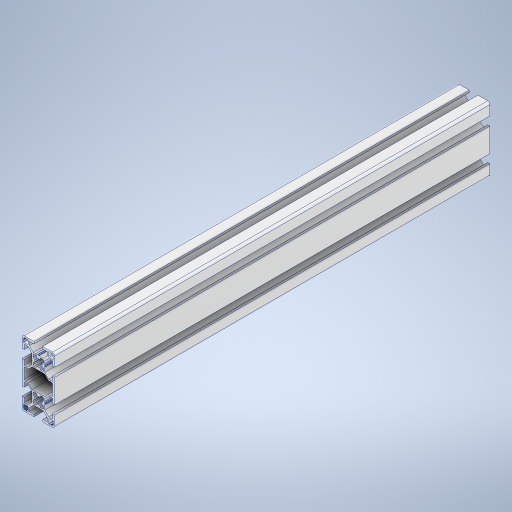
# Autodesk Inventor part: NFSL6-3060-700
Saved by Autodesk Inventor 2024 (Build 280153000, 153)
## iProperties
Category: PARTsolutions
Company: MISUMI
Created: 2024-12-13
Part Number: NFSL6-3060-700
Material: アルミニウム 6061
Catalog Web Link: www.cadenas.de
Description: NEFS6-3060, NEFSB6-3060, NEFSY6-3060, EFS6-3060, EFSB6-3060, HFS6-3060, HFSB6-3060, CAF6-3060, NFSL6-3060, HFSL6-3060, HFSLB6-3060, GFS6-3060, HFSY6-3060-Aluminum Frames -6 Series-2 Row Groove 30x60 mm Square-Specified Length
Vendor: MISUMI
Document SubType Name: Modeling
Designer: psAdmin
Manufacturer: MISUMI
Mass: 914.122 g
Surface Area: 4208.9 cm^2
Volume: 338.564 cm^3
Density: 2.7 g/cm^3
Appearance: アルミニウム - フラット
PSOL_IDENT_0: {$CADENAS_DATA/23d-libs/misumi/metric/38_al_extrusions_blackets/6/hfs6_3060.prj},757 {VTYP=3D},{NB=N
PSOL_IDENT_1: FSL6-3060-700},{LINA=NFSL6-3060-700},{NN=NEFS6-3060, NEFSB6-3060, NEFSY6-3060, EFS6-3060, EFSB6-3060
PSOL_IDENT_2: , HFS6-3060, HFSB6-3060, CAF6-3060, NFSL6-3060, HFSL6-3060, HFSLB6-3060, GFS6-3060, HFSY6-3060},{DAT
PSOL_IDENT_3: E=31.01.2024 10:05:17},{GEOMDATE=26.07.2023 02:49:00},{VERSION=},{LINEID=80},{WBVAR=L,ALT1,ALT2,ALT3
PSOL_IDENT_4: ,ALT4,ALT5,CP5,DL5,DR5,ALT6,ALT9,ALT10,ALT11,DD6SE,DD6,HP6,NHL6,DL6,NHR6,DR6,ALT7,ALT8,NH9,AH,BH,CH,
PSOL_IDENT_5: DH,EH,NH10,AV,BV,CV,DV,EV,NH11,AP,BP,CP,DP,EP,ALT12,ALT13,Z,NH12,XA,XB,XC,XD,XE,NH13,YA,YB,YC,YD,YE,
PSOL_IDENT_6: ALT14,HP14,DL14,DR14,ALT15,HP15,DL15,DR15,ALT16,HP16,DL16,DR16,ALT17,HQ17,JLP,ALT18,HQ18,KLP,ALT19,A
PSOL_IDENT_7: LT20},{WBNUMERIC=L,DD6,NH9,AH,BH,CH,DH,EH,NH10,AV,BV,CV,DV,EV,NH11,AP,BP,CP,DP,EP,NH12,XA,XB,XC,XD,X
PSOL_IDENT_8: E,NH13,YA,YB,YC,YD,YE,HQ17,JLP,HQ18,KLP}  {NB=NFSL6-3060-700},{LINA=NFSL6-3060-700},{KT=DUMMY},{PN=N
PSOL_IDENT_9: FSL6-3060-700},{TPS=NFSL6-3060},{MAT=6063-T5 Aluminum Alloy},{ST=Clear Anodize},{FRMW=30},{FRMH=60},
PSOL_IDENT_10: {FRD=6.8},{L=700.0},{MASS=1.29},{SA=476},{LX=4.87x10^4},{LY=17.87x10^4},{ALT1=},{M1=0},{IDM1=6.647},
PSOL_IDENT_11: {DALT1=4.2},{DPL1=0},{DPR1=0},{ALT1PN=},{ALT2=},{ALT2ALG= '','w/o End Tapping (Insert)','LHP','with
PSOL_IDENT_12: LHP (Tapping on the Left (Insert))','RHP','with RHP (Tapping on the Right (Insert))','HPW','with HPW
PSOL_IDENT_13: (Tapping on Both Ends (Insert))' },{M2=0},{DP2=0},{ALT2PN=},{ALT3=},{ALT3ALG= '','N/A' },{M3=0},{ID
PSOL_IDENT_14: M3=4.134},{DP3=0},{ALT3PN=},{ALT4=},{ALT4ALG= '', 'w/o SC (High Precision Cut)', 'SC', 'with SC (Hig
PSOL_IDENT_15: h Precision Cut)' },{ALT4PN=},{ALT5=},{ALT5ALG= '','w/o 45 Degree Cut','1','with 45 Degree Cut' },{C
PSOL_IDENT_16: P5=},{CP5ALG= '','N/A' },{DL5=},{DL5ALG= '','N/A' },{DR5=},{DR5ALG= '','N/A' },{FRMLALT5=0},{FRMRALT
PSOL_IDENT_17: 5=0},{ALT5PN=},{ALT6=},{ALT6ALG= '','w/o Fastening Location Wrench Access Hole Alterations','1','wit
PSOL_IDENT_18: h Fastening Location Wrench Access Hole Alterations' },{ALT9=},{ALT9ALG= '','w/o Location Specified
PSOL_IDENT_19: Wrench Access Hole Alteratons (Horizontal)','1','with Location Specified Wrench Access Hole Alterato
PSOL_IDENT_20: ns (Horizontal)' },{ALT10=},{ALT10ALG= '','w/o Location Specified Wrench Access Hole Alteratons (Ver
PSOL_IDENT_21: tical)','1','with Location Specified Wrench Access Hole Alteratons (Vertical)' },{ALT11=},{ALT11ALG=
PSOL_IDENT_22: '','w/o Location Specified Wrench Access Hole Alteratons (Crisscross)','1','with Location Specified
PSOL_IDENT_23: Wrench Access Hole Alteratons (Crisscross)' },{DD6SE=},{DD6SEALG= '','N/A' },{DD6=0},{DD6ALG=0},{HP
PSOL_IDENT_24: 6=},{HP6ALG= '','N/A' },{NHL6=},{NHL6ALG= '','N/A' },{DL6=},{DL6ALG= '','N/A' },{NHR6=},{NHR6ALG= ''
PSOL_IDENT_25: ,'N/A' },{DR6=},{DR6ALG= '','N/A' },{DD6PN=},{HL6=0},{HL6D=0},{HR6=0},{HR6D=0},{J6=0},{J6D=0},{K6=0}
PSOL_IDENT_26: ,{K6D=0},{ALT7=},{ALT7ALG= '','N/A' },{ALT8=},{ALT8ALG= '','N/A' },{ALT678PN=},{NH9=0},{NH9MAX=5},{N
PSOL_IDENT_27: H9ALG=[0]},{AH=0.0},{AHMIN=7},{AHMAX=695},{AHALG=[0]},{BH=0.0},{BHMIN=2},{BHMAX=697},{BHALG=[0]},{CH=
PSOL_IDENT_28: 0.0},{CHMIN=2},{CHMAX=699},{CHALG=[0]},{DH=0.0},{DHMIN=2},{DHMAX=701},{DHALG=[0]},{EH=0.0},{EHMIN=2}
PSOL_IDENT_29: ,{EHMAX=693},{EHALG=[0]},{NH10=0},{NH10MAX=5},{NH10ALG=[0]},{AV=0.0},{AVMIN=7},{AVMAX=695},{AVALG=[0
PSOL_IDENT_30: ]},{BV=0.0},{BVMIN=2},{BVMAX=697},{BVALG=[0]},{CV=0.0},{CVMIN=2},{CVMAX=699},{CVALG=[0]},{DV=0.0},{D
PSOL_IDENT_31: VMIN=2},{DVMAX=701},{DVALG=[0]},{EV=0.0},{EVMIN=2},{EVMAX=693},{EVALG=[0]},{NH11=0},{NH11MAX=5},{NH1
PSOL_IDENT_32: 1ALG=[0]},{AP=0.0},{APMIN=7},{APMAX=695},{APALG=[0]},{BP=0.0},{BPMIN=2},{BPMAX=697},{BPALG=[0]},{CP=
PSOL_IDENT_33: 0.0},{CPMIN=2},{CPMAX=699},{CPALG=[0]},{DP=0.0},{DPMIN=2},{DPMAX=701},{DPALG=[0]},{EP=0.0},{EPMIN=2}
PSOL_IDENT_34: ,{EPMAX=693},{EPALG=[0]},{ALT9PN=},{ALT10PN=},{ALT11PN=},{ALT91011PN=},{ALT12=},{ALT12ALG= '','w/o C
PSOL_IDENT_35: ounterbore Hole in Specified Position (Vertical)','1','with Counterbore Hole in Specified Position (
PSOL_IDENT_36: Vertical)' },{ALT13=},{ALT13ALG= '','w/o Counterbore Hole in Specified Position (Horizontal)','1','w
PSOL_IDENT_37: ith Counterbore Hole in Specified Position (Horizontal)' },{Z=},{ZALG= '','N/A' },{DD12=0.0},{DD112=
PSOL_IDENT_38: 0.0},{NH12=0},{NH12MAX=5},{NH12ALG=[0]},{XA=0.0},{XAMIN=7},{XAMAX=695},{XAALG=[0]},{XB=0.0},{XBMIN=2
PSOL_IDENT_39: },{XBMAX=697},{XBALG=[0]},{XC=0.0},{XCMIN=2},{XCMAX=699},{XCALG=[0]},{XD=0.0},{XDMIN=2},{XDMAX=701},
PSOL_IDENT_40: {XDALG=[0]},{XE=0.0},{XEMIN=2},{XEMAX=693},{XEALG=[0]},{NH13=0},{NH13MAX=5},{NH13ALG=[0]},{YA=0.0},{
PSOL_IDENT_41: YAMIN=7},{YAMAX=695},{YAALG=[0]},{YB=0.0},{YBMIN=2},{YBMAX=697},{YBALG=[0]},{YC=0.0},{YCMIN=2},{YCMA
PSOL_IDENT_42: X=699},{YCALG=[0]},{YD=0.0},{YDMIN=2},{YDMAX=701},{YDALG=[0]},{YE=0.0},{YEMIN=2},{YEMAX=693},{YEALG=
PSOL_IDENT_43: [0]},{ALT12PN=},{ALT13PN=},{ALT1213PN=},{ALT14=},{ALT14ALG= '','w/o D Type Hole Alteration','1','wit
PSOL_IDENT_44: h D Type Hole Alteration' },{HP14=},{HP14ALG= '','N/A' },{DL14=},{DL14ALG= '','N/A' },{DR14=},{DR14A
PSOL_IDENT_45: LG= '','N/A' },{H14=0},{D14=0.0},{ALT14PN=},{ALT15=},{ALT15ALG= '','w/o S Type Hole Alteration','1','
PSOL_IDENT_46: with S Type Hole Alteration' },{HP15=},{HP15ALG= '','N/A' },{DL15=},{DL15ALG= '','N/A' },{DR15=},{DR
PSOL_IDENT_47: 15ALG= '','N/A' },{H15=0},{D115=0.0},{D215=0.0},{ALT15PN=},{ALT16=},{ALT16ALG= '','w/o M Type Hole A
PSOL_IDENT_48: lteration','1','with M Type Hole Alteration' },{HP16=},{HP16ALG= '','N/A' },{DL16=},{DL16ALG= '','N/
PSOL_IDENT_49: A' },{DR16=},{DR16ALG= '','N/A' },{H116=0},{D16=0.0},{ALT16PN=},{ALT17=},{ALT17ALG= '','w/o L Type H
PSOL_IDENT_50: ole Alteration (Top)','1','with L Type Hole Alteration (Top)' },{HQ17=0},{HQ17ALG=0},{JLP=0},{JLPMIN=
PSOL_IDENT_51: 4.9},{JLPMAX=0},{JLPALG=[0]},{L17=0},{D17=0.0},{ALT18=},{ALT18ALG= '','w/o L Type Hole Alteration (B
PSOL_IDENT_52: ottom)','1','with L Type Hole Alteration (Bottom)' },{HQ18=0},{HQ18ALG=0},{KLP=0},{KLPALG=[0]},{KLPM
PSOL_IDENT_53: IN=4.9},{KLPMAX=0},{L18=0},{D18=0.0},{ALT19=},{ALT19ALG= '','N/A' },{M19=0},{DP19=0},{ALT1718PN=},{A
PSOL_IDENT_54: LT19PN=},{ALT20=},{ALT20PN=},{ERRORALT01=OK},{ERRORALT02=OK},{ERRORALT03=OK},{ERRORALT05=OK},{ERRORA
PSOL_IDENT_55: LT06091=OK},{ERRORALT06092=OK},{ERRORALT06093=OK},{ERRORALT06094=OK},{ERRORALT06101=OK},{ERRORALT061
PSOL_IDENT_56: 02=OK},{ERRORALT06103=OK},{ERRORALT06104=OK},{ERRORALT06111=OK},{ERRORALT06112=OK},{ERRORALT06113=OK
PSOL_IDENT_57: },{ERRORALT06114=OK},{ERRORALT06121=OK},{ERRORALT06122=OK},{ERRORALT06123=OK},{ERRORALT06124=OK},{ER
PSOL_IDENT_58: RORALT06131=OK},{ERRORALT06132=OK},{ERRORALT06133=OK},{ERRORALT06134=OK},{ERRORALT0614=OK},{ERRORALT
PSOL_IDENT_59: 0615=OK},{ERRORALT0616=OK},{ERRORALT06171=OK},{ERRORALT06172=OK},{ERRORALT06173=OK},{ERRORALT06181=O
PSOL_IDENT_60: K},{ERRORALT06182=OK},{ERRORALT06183=OK},{ERRORALT0619=OK},{ERRORALT0911=OK},{ERRORALT0913=OK},{ERRO
PSOL_IDENT_61: RALT0914=OK},{ERRORALT0915=OK},{ERRORALT0916=OK},{ERRORALT0917=OK},{ERRORALT0918=OK},{ERRORALT0919=O
PSOL_IDENT_62: K},{ERRORALT1011=OK},{ERRORALT1012=OK},{ERRORALT1014=OK},{ERRORALT1015=OK},{ERRORALT1016=OK},{ERRORA
PSOL_IDENT_63: LT1017=OK},{ERRORALT1018=OK},{ERRORALT1019=OK},{ERRORALT1112=OK},{ERRORALT1113=OK},{ERRORALT1114=OK}
PSOL_IDENT_64: ,{ERRORALT1115=OK},{ERRORALT1116=OK},{ERRORALT1117=OK},{ERRORALT1118=OK},{ERRORALT1119=OK},{ERRORALT
PSOL_IDENT_65: 1214=OK},{ERRORALT1215=OK},{ERRORALT1216=OK},{ERRORALT1217=OK},{ERRORALT1218=OK},{ERRORALT1219=OK},{
PSOL_IDENT_66: ERRORALT1314=OK},{ERRORALT1315=OK},{ERRORALT1316=OK},{ERRORALT1317=OK},{ERRORALT1318=OK},{ERRORALT13
PSOL_IDENT_67: 19=OK},{ERRORALT1415=OK},{ERRORALT1416=OK},{ERRORALT1417=OK},{ERRORALT1418=OK},{ERRORALT1419=OK},{ER
PSOL_IDENT_68: RORALT1516=OK},{ERRORALT1517=OK},{ERRORALT1518=OK},{ERRORALT1519=OK},{ERRORALT1617=OK},{ERRORALT1618=
PSOL_IDENT_69: OK},{ERRORALT1619=OK},{ERRORALT1719=OK},{ERRORALT1819=OK},{ERRORPN=},{COLOR=}
NB: NFSL6-3060-700
NN: NEFS6-3060, NEFSB6-3060, NEFSY6-3060, EFS6-3060, EFSB6-3060, HFS6-3060, HFSB6-3060, CAF6-3060, NFSL6-3060, HFSL6-3060, HFSLB6-3060, GFS6-3060, HFSY6-3060
NT: Aluminum Frames -6 Series-2 Row Groove 30x60 mm Square-Specified Length
NBSYN: $PN.
LINA: NFSL6-3060-700
CATALOG: Misumi
PN: NFSL6-3060-700
TPS: NFSL6-3060
MAT: 6063-T5 Aluminum Alloy
ST: Clear Anodize
L: 700
MASS: 1.29
SA: 476
LX: 4.87x10^4
LY: 17.87x10^4
ALT1: w/o End Tapping
DPL1: 0
DPR1: 0
ALT2: w/o End Tapping (Insert)
M2: 0
DP2: 0
ALT3: N/A
M3: 0
DP3: 0
ALT4: w/o SC (High Precision Cut)
ALT5: w/o 45 Degree Cut
CP5: N/A
DL5: N/A
DR5: N/A
ALT6: w/o Fastening Location Wrench Access Hole Alterations
ALT9: w/o Location Specified Wrench Access Hole Alteratons (Horizontal)
ALT10: w/o Location Specified Wrench Access Hole Alteratons (Vertical)
ALT11: w/o Location Specified Wrench Access Hole Alteratons (Crisscross)
DD6SE: N/A
DD6: 0
HP6: N/A
NHL6: N/A
DL6: N/A
NHR6: N/A
DR6: N/A
HL6D: 0
HR6D: 0
J6D: 0
K6D: 0
ALT7: N/A
ALT8: N/A
NH9: 0
AH: 0
BH: 0
CH: 0
DH: 0
EH: 0
NH10: 0
AV: 0
BV: 0
CV: 0
DV: 0
EV: 0
NH11: 0
AP: 0
BP: 0
CP: 0
DP: 0
EP: 0
ALT12: w/o Counterbore Hole in Specified Position (Vertical)
ALT13: w/o Counterbore Hole in Specified Position (Horizontal)
Z: N/A
DD12: 0
DD112: 0
NH12: 0
XA: 0
XB: 0
XC: 0
XD: 0
XE: 0
NH13: 0
YA: 0
YB: 0
YC: 0
YD: 0
YE: 0
ALT14: w/o D Type Hole Alteration
HP14: N/A
DL14: N/A
DR14: N/A
H14: 0
D14: 0
ALT15: w/o S Type Hole Alteration
HP15: N/A
DL15: N/A
DR15: N/A
H15: 0
D115: 0
D215: 0
ALT16: w/o M Type Hole Alteration
HP16: N/A
DL16: N/A
DR16: N/A
H116: 0
D16: 0
ALT17: w/o L Type Hole Alteration (Top)
HQ17: 0
JLP: 0
D17: 0
ALT18: w/o L Type Hole Alteration (Bottom)
HQ18: 0
KLP: 0
D18: 0
ALT19: N/A
M19: 0
DP19: 0
ALT20: w/o CW (End Face C Chamfering)
SUPPLIER: MISUMI
ARTICLENO: NFSL6-3060-700
BOMINFO: NFSL6-3060-700
CREATOR: CADENAS GmbH
Title: NFSL6-3060-700
Author: Cadenas PARTsolutions
Comments: Aluminum Frames -6 Series-2 Row Groove 30x60 mm Square-Specified Length
Autodesk Inventor part; units mm, degrees
sketch "Sketch_118" plane through (0, 0, 0) normal (0, 0, 1) x (1, 0, 0)
  line L0 (-15, 11) -> (-15, -11)
  line L1 (-15, -11) -> (-13, -11)
  line L2 (-13, -11) -> (-13, -6.75)
  line L3 (-13, -6.75) -> (-9.6642, -6.75)
  line L4 (-9.6642, -6.75) -> (-6, -10.4142)
  line L5 (-6, -10.4142) -> (-6, -14.3464)
  arc A0 (-6, -14.3464) -> (-5.933, -14.5964) centre (-5.5, -14.3464) ccw
  line L6 (-5.933, -14.5964) -> (-5.7, -15)
  line L7 (-5.7, -15) -> (-5.933, -15.4036)
  arc A1 (-5.933, -15.4036) -> (-5.933, -15.9036) centre (-5.5, -15.6536) ccw
  line L8 (-5.933, -15.9036) -> (-5.751, -16.2189)
  line L9 (-5.751, -16.2189) -> (-6, -17.5)
  line L10 (-6, -17.5) -> (-6, -19.5858)
  line L11 (-6, -19.5858) -> (-9.6642, -23.25)
  line L12 (-9.6642, -23.25) -> (-13, -23.25)
  line L13 (-13, -23.25) -> (-13, -19)
  line L14 (-13, -19) -> (-15, -19)
  line L15 (-15, -19) -> (-15, -28)
  arc A2 (-15, -28) -> (-13, -30) centre (-13, -28) ccw
  line L16 (-13, -30) -> (-4, -30)
  line L17 (-4, -30) -> (-4, -28)
  line L18 (-4, -28) -> (-8.25, -28)
  line L19 (-8.25, -28) -> (-8.25, -24.6642)
  line L20 (-8.25, -24.6642) -> (-4.5858, -21)
  line L21 (-4.5858, -21) -> (-0.6536, -21)
  arc A3 (-0.6536, -21) -> (-0.4036, -20.933) centre (-0.6536, -20.5) ccw
  line L22 (-0.4036, -20.933) -> (0, -20.7)
  line L23 (0, -20.7) -> (0.4036, -20.933)
  arc A4 (0.4036, -20.933) -> (0.9036, -20.933) centre (0.6536, -20.5) ccw
  line L24 (0.9036, -20.933) -> (1.2189, -20.751)
  line L25 (1.2189, -20.751) -> (2.5, -21)
  line L26 (2.5, -21) -> (4.5858, -21)
  line L27 (4.5858, -21) -> (8.25, -24.6642)
  line L28 (8.25, -24.6642) -> (8.25, -28)
  line L29 (8.25, -28) -> (4, -28)
  line L30 (4, -28) -> (4, -30)
  line L31 (4, -30) -> (13, -30)
  arc A5 (13, -30) -> (15, -28) centre (13, -28) ccw
  line L32 (15, -28) -> (15, -19)
  line L33 (15, -19) -> (13, -19)
  line L34 (13, -19) -> (13, -23.25)
  line L35 (13, -23.25) -> (9.6642, -23.25)
  line L36 (9.6642, -23.25) -> (6, -19.5858)
  line L37 (6, -19.5858) -> (6, -15.6536)
  arc A6 (6, -15.6536) -> (5.933, -15.4036) centre (5.5, -15.6536) ccw
  line L38 (5.933, -15.4036) -> (5.7, -15)
  line L39 (5.7, -15) -> (5.933, -14.5964)
  arc A7 (5.933, -14.5964) -> (5.933, -14.0964) centre (5.5, -14.3464) ccw
  line L40 (5.933, -14.0964) -> (5.751, -13.7811)
  line L41 (5.751, -13.7811) -> (6, -12.5)
  line L42 (6, -12.5) -> (6, -10.4142)
  line L43 (6, -10.4142) -> (9.6642, -6.75)
  line L44 (9.6642, -6.75) -> (13, -6.75)
  line L45 (13, -6.75) -> (13, -11)
  line L46 (13, -11) -> (15, -11)
  line L47 (15, -11) -> (15, 11)
  line L48 (15, 11) -> (13, 11)
  line L49 (13, 11) -> (13, 6.75)
  line L50 (13, 6.75) -> (9.6642, 6.75)
  line L51 (9.6642, 6.75) -> (6, 10.4142)
  line L52 (6, 10.4142) -> (6, 14.3464)
  arc A8 (6, 14.3464) -> (5.933, 14.5964) centre (5.5, 14.3464) ccw
  line L53 (5.933, 14.5964) -> (5.7, 15)
  line L54 (5.7, 15) -> (5.933, 15.4036)
  arc A9 (5.933, 15.4036) -> (5.933, 15.9036) centre (5.5, 15.6536) ccw
  line L55 (5.933, 15.9036) -> (5.751, 16.2189)
  line L56 (5.751, 16.2189) -> (6, 17.5)
  line L57 (6, 17.5) -> (6, 19.5858)
  line L58 (6, 19.5858) -> (9.6642, 23.25)
  line L59 (9.6642, 23.25) -> (13, 23.25)
  line L60 (13, 23.25) -> (13, 19)
  line L61 (13, 19) -> (15, 19)
  line L62 (15, 19) -> (15, 28)
  arc A10 (15, 28) -> (13, 30) centre (13, 28) ccw
  line L63 (13, 30) -> (4, 30)
  line L64 (4, 30) -> (4, 28)
  line L65 (4, 28) -> (8.25, 28)
  line L66 (8.25, 28) -> (8.25, 24.6642)
  line L67 (8.25, 24.6642) -> (4.5858, 21)
  line L68 (4.5858, 21) -> (0.6536, 21)
  arc A11 (0.6536, 21) -> (0.4036, 20.933) centre (0.6536, 20.5) ccw
  line L69 (0.4036, 20.933) -> (0, 20.7)
  line L70 (0, 20.7) -> (-0.4036, 20.933)
  arc A12 (-0.4036, 20.933) -> (-0.9036, 20.933) centre (-0.6536, 20.5) ccw
  line L71 (-0.9036, 20.933) -> (-1.2189, 20.751)
  line L72 (-1.2189, 20.751) -> (-2.5, 21)
  line L73 (-2.5, 21) -> (-4.5858, 21)
  line L74 (-4.5858, 21) -> (-8.25, 24.6642)
  line L75 (-8.25, 24.6642) -> (-8.25, 28)
  line L76 (-8.25, 28) -> (-4, 28)
  line L77 (-4, 28) -> (-4, 30)
  line L78 (-4, 30) -> (-13, 30)
  arc A13 (-13, 30) -> (-15, 28) centre (-13, 28) ccw
  line L79 (-15, 28) -> (-15, 19)
  line L80 (-15, 19) -> (-13, 19)
  line L81 (-13, 19) -> (-13, 23.25)
  line L82 (-13, 23.25) -> (-9.6642, 23.25)
  line L83 (-9.6642, 23.25) -> (-6, 19.5858)
  line L84 (-6, 19.5858) -> (-6, 15.6536)
  arc A14 (-6, 15.6536) -> (-5.933, 15.4036) centre (-5.5, 15.6536) ccw
  line L85 (-5.933, 15.4036) -> (-5.7, 15)
  line L86 (-5.7, 15) -> (-5.933, 14.5964)
  arc A15 (-5.933, 14.5964) -> (-5.933, 14.0964) centre (-5.5, 14.3464) ccw
  line L87 (-5.933, 14.0964) -> (-5.751, 13.7811)
  line L88 (-5.751, 13.7811) -> (-6, 12.5)
  line L89 (-6, 12.5) -> (-6, 10.4142)
  line L90 (-6, 10.4142) -> (-9.6642, 6.75)
  line L91 (-9.6642, 6.75) -> (-13, 6.75)
  line L92 (-13, 6.75) -> (-13, 11)
  line L93 (-13, 11) -> (-15, 11)
  line L94 (9.5, 28.6) -> (9.5, 25)
  arc A16 (9.5, 25) -> (10, 24.5) centre (10, 25) ccw
  line L95 (10, 24.5) -> (13.6, 24.5)
  arc A17 (13.6, 24.5) -> (13.8, 24.7) centre (13.6, 24.7) ccw
  line L96 (13.8, 24.7) -> (13.8, 26.2)
  arc A18 (13.8, 26.2) -> (13.6, 26.4) centre (13.6, 26.2) ccw
  line L97 (13.6, 26.4) -> (13.43, 26.4)
  arc A19 (13.23, 26.6) -> (13.43, 26.4) centre (13.43, 26.6) ccw
  line L98 (13.23, 26.6) -> (13.23, 27)
  arc A20 (13.43, 27.2) -> (13.23, 27) centre (13.43, 27) ccw
  line L99 (13.43, 27.2) -> (13.6, 27.2)
  arc A21 (13.6, 27.2) -> (13.8, 27.4) centre (13.6, 27.4) ccw
  line L100 (13.8, 27.4) -> (13.8, 27.6)
  arc A22 (13.8, 27.6) -> (13.5, 27.9) centre (13.5, 27.6) ccw
  line L101 (13.5, 27.9) -> (13.2, 27.9)
  arc A23 (12.9, 28.2) -> (13.2, 27.9) centre (13.2, 28.2) ccw
  line L102 (12.9, 28.2) -> (12.9, 28.5)
  arc A24 (12.9, 28.5) -> (12.6, 28.8) centre (12.6, 28.5) ccw
  line L103 (12.6, 28.8) -> (12.4, 28.8)
  arc A25 (12.4, 28.8) -> (12.2, 28.6) centre (12.4, 28.6) ccw
  line L104 (12.2, 28.6) -> (12.2, 28.43)
  arc A26 (12, 28.23) -> (12.2, 28.43) centre (12, 28.43) ccw
  line L105 (12, 28.23) -> (11.6, 28.23)
  arc A27 (11.4, 28.43) -> (11.6, 28.23) centre (11.6, 28.43) ccw
  line L106 (11.4, 28.43) -> (11.4, 28.6)
  arc A28 (11.4, 28.6) -> (11.2, 28.8) centre (11.2, 28.6) ccw
  line L107 (11.2, 28.8) -> (9.7, 28.8)
  arc A29 (9.7, 28.8) -> (9.5, 28.6) centre (9.7, 28.6) ccw
  arc A30 (9.5, -28.6) -> (9.7, -28.8) centre (9.7, -28.6) ccw
  line L108 (9.7, -28.8) -> (11.2, -28.8)
  arc A31 (11.2, -28.8) -> (11.4, -28.6) centre (11.2, -28.6) ccw
  line L109 (11.4, -28.6) -> (11.4, -28.43)
  arc A32 (11.6, -28.23) -> (11.4, -28.43) centre (11.6, -28.43) ccw
  line L110 (11.6, -28.23) -> (12, -28.23)
  arc A33 (12.2, -28.43) -> (12, -28.23) centre (12, -28.43) ccw
  line L111 (12.2, -28.43) -> (12.2, -28.6)
  arc A34 (12.2, -28.6) -> (12.4, -28.8) centre (12.4, -28.6) ccw
  line L112 (12.4, -28.8) -> (12.6, -28.8)
  arc A35 (12.6, -28.8) -> (12.9, -28.5) centre (12.6, -28.5) ccw
  line L113 (12.9, -28.5) -> (12.9, -28.2)
  arc A36 (13.2, -27.9) -> (12.9, -28.2) centre (13.2, -28.2) ccw
  line L114 (13.2, -27.9) -> (13.5, -27.9)
  arc A37 (13.5, -27.9) -> (13.8, -27.6) centre (13.5, -27.6) ccw
  line L115 (13.8, -27.6) -> (13.8, -27.4)
  arc A38 (13.8, -27.4) -> (13.6, -27.2) centre (13.6, -27.4) ccw
  line L116 (13.6, -27.2) -> (13.43, -27.2)
  arc A39 (13.23, -27) -> (13.43, -27.2) centre (13.43, -27) ccw
  line L117 (13.23, -27) -> (13.23, -26.6)
  arc A40 (13.43, -26.4) -> (13.23, -26.6) centre (13.43, -26.6) ccw
  line L118 (13.43, -26.4) -> (13.6, -26.4)
  arc A41 (13.6, -26.4) -> (13.8, -26.2) centre (13.6, -26.2) ccw
  line L119 (13.8, -26.2) -> (13.8, -24.7)
  arc A42 (13.8, -24.7) -> (13.6, -24.5) centre (13.6, -24.7) ccw
  line L120 (13.6, -24.5) -> (10, -24.5)
  arc A43 (10, -24.5) -> (9.5, -25) centre (10, -25) ccw
  line L121 (9.5, -25) -> (9.5, -28.6)
  arc A44 (-13, -4.55) -> (-12, -5.55) centre (-12, -4.55) ccw
  line L122 (-12, -5.55) -> (-9.1672, -5.55)
  line L123 (-9.1672, -5.55) -> (-5.7172, -9)
  line L124 (-5.7172, -9) -> (5.7172, -9)
  line L125 (5.7172, -9) -> (9.1672, -5.55)
  line L126 (9.1672, -5.55) -> (12, -5.55)
  arc A45 (12, -5.55) -> (13, -4.55) centre (12, -4.55) ccw
  line L127 (13, -4.55) -> (13, 4.55)
  arc A46 (13, 4.55) -> (12, 5.55) centre (12, 4.55) ccw
  line L128 (12, 5.55) -> (9.1672, 5.55)
  line L129 (9.1672, 5.55) -> (5.7172, 9)
  line L130 (5.7172, 9) -> (-5.7172, 9)
  line L131 (-5.7172, 9) -> (-9.1672, 5.55)
  line L132 (-9.1672, 5.55) -> (-12, 5.55)
  arc A47 (-12, 5.55) -> (-13, 4.55) centre (-12, 4.55) ccw
  line L133 (-13, 4.55) -> (-13, -4.55)
  line L134 (-13.8, 26.2) -> (-13.8, 24.7)
  arc A48 (-13.8, 24.7) -> (-13.6, 24.5) centre (-13.6, 24.7) ccw
  line L135 (-13.6, 24.5) -> (-10, 24.5)
  arc A49 (-10, 24.5) -> (-9.5, 25) centre (-10, 25) ccw
  line L136 (-9.5, 25) -> (-9.5, 28.6)
  arc A50 (-9.5, 28.6) -> (-9.7, 28.8) centre (-9.7, 28.6) ccw
  line L137 (-9.7, 28.8) -> (-11.2, 28.8)
  arc A51 (-11.2, 28.8) -> (-11.4, 28.6) centre (-11.2, 28.6) ccw
  line L138 (-11.4, 28.6) -> (-11.4, 28.43)
  arc A52 (-11.6, 28.23) -> (-11.4, 28.43) centre (-11.6, 28.43) ccw
  line L139 (-11.6, 28.23) -> (-12, 28.23)
  arc A53 (-12.2, 28.43) -> (-12, 28.23) centre (-12, 28.43) ccw
  line L140 (-12.2, 28.43) -> (-12.2, 28.6)
  arc A54 (-12.2, 28.6) -> (-12.4, 28.8) centre (-12.4, 28.6) ccw
  line L141 (-12.4, 28.8) -> (-12.6, 28.8)
  arc A55 (-12.6, 28.8) -> (-12.9, 28.5) centre (-12.6, 28.5) ccw
  line L142 (-12.9, 28.5) -> (-12.9, 28.2)
  arc A56 (-13.2, 27.9) -> (-12.9, 28.2) centre (-13.2, 28.2) ccw
  line L143 (-13.2, 27.9) -> (-13.5, 27.9)
  arc A57 (-13.5, 27.9) -> (-13.8, 27.6) centre (-13.5, 27.6) ccw
  line L144 (-13.8, 27.6) -> (-13.8, 27.4)
  arc A58 (-13.8, 27.4) -> (-13.6, 27.2) centre (-13.6, 27.4) ccw
  line L145 (-13.6, 27.2) -> (-13.43, 27.2)
  arc A59 (-13.23, 27) -> (-13.43, 27.2) centre (-13.43, 27) ccw
  line L146 (-13.23, 27) -> (-13.23, 26.6)
  arc A60 (-13.43, 26.4) -> (-13.23, 26.6) centre (-13.43, 26.6) ccw
  line L147 (-13.43, 26.4) -> (-13.6, 26.4)
  arc A61 (-13.6, 26.4) -> (-13.8, 26.2) centre (-13.6, 26.2) ccw
  arc A62 (-13.8, -26.2) -> (-13.6, -26.4) centre (-13.6, -26.2) ccw
  line L148 (-13.6, -26.4) -> (-13.43, -26.4)
  arc A63 (-13.23, -26.6) -> (-13.43, -26.4) centre (-13.43, -26.6) ccw
  line L149 (-13.23, -26.6) -> (-13.23, -27)
  arc A64 (-13.43, -27.2) -> (-13.23, -27) centre (-13.43, -27) ccw
  line L150 (-13.43, -27.2) -> (-13.6, -27.2)
  arc A65 (-13.6, -27.2) -> (-13.8, -27.4) centre (-13.6, -27.4) ccw
  line L151 (-13.8, -27.4) -> (-13.8, -27.6)
  arc A66 (-13.8, -27.6) -> (-13.5, -27.9) centre (-13.5, -27.6) ccw
  line L152 (-13.5, -27.9) -> (-13.2, -27.9)
  arc A67 (-12.9, -28.2) -> (-13.2, -27.9) centre (-13.2, -28.2) ccw
  line L153 (-12.9, -28.2) -> (-12.9, -28.5)
  arc A68 (-12.9, -28.5) -> (-12.6, -28.8) centre (-12.6, -28.5) ccw
  line L154 (-12.6, -28.8) -> (-12.4, -28.8)
  arc A69 (-12.4, -28.8) -> (-12.2, -28.6) centre (-12.4, -28.6) ccw
  line L155 (-12.2, -28.6) -> (-12.2, -28.43)
  arc A70 (-12, -28.23) -> (-12.2, -28.43) centre (-12, -28.43) ccw
  line L156 (-12, -28.23) -> (-11.6, -28.23)
  arc A71 (-11.4, -28.43) -> (-11.6, -28.23) centre (-11.6, -28.43) ccw
  line L157 (-11.4, -28.43) -> (-11.4, -28.6)
  arc A72 (-11.4, -28.6) -> (-11.2, -28.8) centre (-11.2, -28.6) ccw
  line L158 (-11.2, -28.8) -> (-9.7, -28.8)
  arc A73 (-9.7, -28.8) -> (-9.5, -28.6) centre (-9.7, -28.6) ccw
  line L159 (-9.5, -28.6) -> (-9.5, -25)
  arc A74 (-9.5, -25) -> (-10, -24.5) centre (-10, -25) ccw
  line L160 (-10, -24.5) -> (-13.6, -24.5)
  arc A75 (-13.6, -24.5) -> (-13.8, -24.7) centre (-13.6, -24.7) ccw
  line L161 (-13.8, -24.7) -> (-13.8, -26.2)
  constraints: 324 end point, 152 point on circle, 76 centre point
extrude "Extrusion1" add sketch "Sketch_118" against normal blind 400
sketch "Sketch_94" plane through (0, 0, 0) normal (0, 0, 1) x (1, 0, 0)
  line L0 (-4.8, 18.8) -> (-4.8, 17.2312)
  arc A0 (-4.8, 17.2312) -> (-4.4833, 16.766) centre (-4.3, 17.2312) ccw
  line L1 (-4.4833, 16.766) -> (-3.5987, 16.4176)
  arc A1 (-3.2971, 15.8303) -> (-3.5987, 16.4176) centre (-3.7819, 15.9524) ccw
  arc A2 (-3.2971, 15.8303) -> (-3.4, 15) centre (0, 15) ccw
  arc A3 (-3.4, 15) -> (-3.2971, 14.1697) centre (0, 15) ccw
  arc A4 (-3.5987, 13.5824) -> (-3.2971, 14.1697) centre (-3.7819, 14.0476) ccw
  line L2 (-3.5987, 13.5824) -> (-4.4833, 13.234)
  arc A5 (-4.4833, 13.234) -> (-4.8, 12.7688) centre (-4.3, 12.7688) ccw
  line L3 (-4.8, 12.7688) -> (-4.8, 11.2)
  arc A6 (-4.8, 11.2) -> (-3.8, 10.2) centre (-3.8, 11.2) ccw
  line L4 (-3.8, 10.2) -> (-2.2312, 10.2)
  arc A7 (-2.2312, 10.2) -> (-1.766, 10.5167) centre (-2.2312, 10.7) ccw
  line L5 (-1.766, 10.5167) -> (-1.4176, 11.4013)
  arc A8 (-0.8303, 11.7029) -> (-1.4176, 11.4013) centre (-0.9524, 11.2181) ccw
  arc A9 (-0.8303, 11.7029) -> (0, 11.6) centre (0, 15) ccw
  arc A10 (0, 11.6) -> (0.8303, 11.7029) centre (0, 15) ccw
  arc A11 (1.4176, 11.4013) -> (0.8303, 11.7029) centre (0.9524, 11.2181) ccw
  line L6 (1.4176, 11.4013) -> (1.766, 10.5167)
  arc A12 (1.766, 10.5167) -> (2.2312, 10.2) centre (2.2312, 10.7) ccw
  line L7 (2.2312, 10.2) -> (3.8, 10.2)
  arc A13 (3.8, 10.2) -> (4.8, 11.2) centre (3.8, 11.2) ccw
  line L8 (4.8, 11.2) -> (4.8, 12.7688)
  arc A14 (4.8, 12.7688) -> (4.4833, 13.234) centre (4.3, 12.7688) ccw
  line L9 (4.4833, 13.234) -> (3.5987, 13.5824)
  arc A15 (3.2971, 14.1697) -> (3.5987, 13.5824) centre (3.7819, 14.0476) ccw
  arc A16 (3.2971, 14.1697) -> (3.4, 15) centre (0, 15) ccw
  arc A17 (3.4, 15) -> (3.2971, 15.8303) centre (0, 15) ccw
  arc A18 (3.5987, 16.4176) -> (3.2971, 15.8303) centre (3.7819, 15.9524) ccw
  line L10 (3.5987, 16.4176) -> (4.4833, 16.766)
  arc A19 (4.4833, 16.766) -> (4.8, 17.2312) centre (4.3, 17.2312) ccw
  line L11 (4.8, 17.2312) -> (4.8, 18.8)
  arc A20 (4.8, 18.8) -> (3.8, 19.8) centre (3.8, 18.8) ccw
  line L12 (3.8, 19.8) -> (2.2312, 19.8)
  arc A21 (2.2312, 19.8) -> (1.766, 19.4833) centre (2.2312, 19.3) ccw
  line L13 (1.766, 19.4833) -> (1.4176, 18.5987)
  arc A22 (0.8303, 18.2971) -> (1.4176, 18.5987) centre (0.9524, 18.7819) ccw
  arc A23 (0.8303, 18.2971) -> (0, 18.4) centre (0, 15) ccw
  arc A24 (0, 18.4) -> (-0.8303, 18.2971) centre (0, 15) ccw
  arc A25 (-1.4176, 18.5987) -> (-0.8303, 18.2971) centre (-0.9524, 18.7819) ccw
  line L14 (-1.4176, 18.5987) -> (-1.766, 19.4833)
  arc A26 (-1.766, 19.4833) -> (-2.2312, 19.8) centre (-2.2312, 19.3) ccw
  line L15 (-2.2312, 19.8) -> (-3.8, 19.8)
  arc A27 (-3.8, 19.8) -> (-4.8, 18.8) centre (-3.8, 18.8) ccw
  constraints: 56 point on circle, 32 end point, 28 centre point
extrude "Extrusion2" cut sketch "Sketch_94" against normal blind 700
sketch "Sketch_113" plane through (0, 0, 0) normal (0, 0, 1) x (1, 0, 0)
  arc A0 (-4.8, -18.8) -> (-3.8, -19.8) centre (-3.8, -18.8) ccw
  line L0 (-3.8, -19.8) -> (-2.2312, -19.8)
  arc A1 (-2.2312, -19.8) -> (-1.766, -19.4833) centre (-2.2312, -19.3) ccw
  line L1 (-1.766, -19.4833) -> (-1.4176, -18.5987)
  arc A2 (-0.8303, -18.2971) -> (-1.4176, -18.5987) centre (-0.9524, -18.7819) ccw
  arc A3 (-0.8303, -18.2971) -> (0, -18.4) centre (0, -15) ccw
  arc A4 (0, -18.4) -> (0.8303, -18.2971) centre (0, -15) ccw
  arc A5 (1.4176, -18.5987) -> (0.8303, -18.2971) centre (0.9524, -18.7819) ccw
  line L2 (1.4176, -18.5987) -> (1.766, -19.4833)
  arc A6 (1.766, -19.4833) -> (2.2312, -19.8) centre (2.2312, -19.3) ccw
  line L3 (2.2312, -19.8) -> (3.8, -19.8)
  arc A7 (3.8, -19.8) -> (4.8, -18.8) centre (3.8, -18.8) ccw
  line L4 (4.8, -18.8) -> (4.8, -17.2312)
  arc A8 (4.8, -17.2312) -> (4.4833, -16.766) centre (4.3, -17.2312) ccw
  line L5 (4.4833, -16.766) -> (3.5987, -16.4176)
  arc A9 (3.2971, -15.8303) -> (3.5987, -16.4176) centre (3.7819, -15.9524) ccw
  arc A10 (3.2971, -15.8303) -> (3.4, -15) centre (0, -15) ccw
  arc A11 (3.4, -15) -> (3.2971, -14.1697) centre (0, -15) ccw
  arc A12 (3.5987, -13.5824) -> (3.2971, -14.1697) centre (3.7819, -14.0476) ccw
  line L6 (3.5987, -13.5824) -> (4.4833, -13.234)
  arc A13 (4.4833, -13.234) -> (4.8, -12.7688) centre (4.3, -12.7688) ccw
  line L7 (4.8, -12.7688) -> (4.8, -11.2)
  arc A14 (4.8, -11.2) -> (3.8, -10.2) centre (3.8, -11.2) ccw
  line L8 (3.8, -10.2) -> (2.2312, -10.2)
  arc A15 (2.2312, -10.2) -> (1.766, -10.5167) centre (2.2312, -10.7) ccw
  line L9 (1.766, -10.5167) -> (1.4176, -11.4013)
  arc A16 (0.8303, -11.7029) -> (1.4176, -11.4013) centre (0.9524, -11.2181) ccw
  arc A17 (0.8303, -11.7029) -> (0, -11.6) centre (0, -15) ccw
  arc A18 (0, -11.6) -> (-0.8303, -11.7029) centre (0, -15) ccw
  arc A19 (-1.4176, -11.4013) -> (-0.8303, -11.7029) centre (-0.9524, -11.2181) ccw
  line L10 (-1.4176, -11.4013) -> (-1.766, -10.5167)
  arc A20 (-1.766, -10.5167) -> (-2.2312, -10.2) centre (-2.2312, -10.7) ccw
  line L11 (-2.2312, -10.2) -> (-3.8, -10.2)
  arc A21 (-3.8, -10.2) -> (-4.8, -11.2) centre (-3.8, -11.2) ccw
  line L12 (-4.8, -11.2) -> (-4.8, -12.7688)
  arc A22 (-4.8, -12.7688) -> (-4.4833, -13.234) centre (-4.3, -12.7688) ccw
  line L13 (-4.4833, -13.234) -> (-3.5987, -13.5824)
  arc A23 (-3.2971, -14.1697) -> (-3.5987, -13.5824) centre (-3.7819, -14.0476) ccw
  arc A24 (-3.2971, -14.1697) -> (-3.4, -15) centre (0, -15) ccw
  arc A25 (-3.4, -15) -> (-3.2971, -15.8303) centre (0, -15) ccw
  arc A26 (-3.5987, -16.4176) -> (-3.2971, -15.8303) centre (-3.7819, -15.9524) ccw
  line L14 (-3.5987, -16.4176) -> (-4.4833, -16.766)
  arc A27 (-4.4833, -16.766) -> (-4.8, -17.2312) centre (-4.3, -17.2312) ccw
  line L15 (-4.8, -17.2312) -> (-4.8, -18.8)
  constraints: 56 point on circle, 32 end point, 28 centre point
extrude "Extrusion3" cut sketch "Sketch_113" against normal blind 700
ref_plane "CP_XY" through (0, 0, -350) normal (1, 0, 0) x (0, 0, -1)
ref_plane "CP_YZ" through (0, 0, -350) normal (0, 0, -1) x (0, 1, 0)
ref_plane "CP_ZX" through (0, 0, -350) normal (0, 1, 0) x (1, 0, 0)
ref_plane "to_frame_cap1_XY" through (0, 15, 0) normal (0, 0, 1) x (1, 0, 0)
ref_plane "to_frame_cap1_YZ" through (0, 15, 0) normal (1, 0, 0) x (0, 1, 0)
ref_plane "to_frame_cap1_ZX" through (0, 15, 0) normal (0, 1, 0) x (0, 0, 1)
ref_plane "to_frame_cap2_XY" through (0, 15, -700) normal (0, 0, -1) x (1, 0, 0)
ref_plane "to_frame_cap2_YZ" through (0, 15, -700) normal (1, 0, 0) x (0, -1, 0)
ref_plane "to_frame_cap2_ZX" through (0, 15, -700) normal (0, -1, 0) x (0, 0, -1)
body "Solid1"
